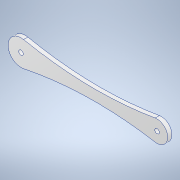
# Autodesk Inventor part: オムニ_支え板
Saved by Autodesk Inventor 2021 (Build 250183000, 183)
## iProperties
Created: 2022-02-03
Part Number: オムニ_支え板
Material: アルミニウム 6061
Document SubType Name: Modeling
Designer: hirohumi
Density: 2.7 g/cm^3
Appearance: アルミニウム - フラット
Author: hirohumi
Autodesk Inventor part; units mm, degrees
ref_plane "YZ Plane" through (0, 0, 0) normal (1, 0, 0) x (0, 1, 0)
ref_plane "XZ Plane" through (0, 0, 0) normal (0, 1, 0) x (-1, 0, 0)
ref_plane "XY Plane" through (0, 0, 0) normal (0, 0, 1) x (1, 0, 0)
sketch "スケッチ1" plane through (0, 0, 0) normal (0, 0, 1) x (1, 0, 0)
  circle A0 centre (-48, 0) radius 1.6
  circle A1 centre (48, 0) radius 1.6
  arc A2 (-46.163, 8.9126) -> (-46.163, -8.9126) centre (-48, 0) ccw
  arc A3 (46.7273, -7.3912) -> (46.7273, 7.3912) centre (48, 0) ccw
  arc A4 (-46.163, 8.9126) -> (46.7273, 7.3912) centre (4.305, 253.7656) ccw
  arc A5 (46.7273, -7.3912) -> (-46.163, -8.9126) centre (4.305, -253.7656) ccw
  point P0 (0, 0)
  dimension "d0" = 3.2
  dimension "d1" = 3.2
  dimension "d2" = 96
  dimension "d3" = 48
  dimension "d4" = 7.5
  dimension "d5" = 7.5
  dimension "d6" = 250
  dimension "d7" = 250
  constraints: 8 point on circle, 6 centre point, 4 tangent, 2 coincident, 2 horizontal alignment
  measures "d0" diameter of A0
  measures "d1" diameter of A1
  measures "d2" distance of A1.centre A0.centre
  measures "d3" distance of point (0, 0) A0.centre
  measures "d4" radial gap between concentric circles of A0 A2
  measures "d5" radius of A3
  measures "d6" radius of A4
  measures "d7" radius of A5
extrude "押し出し1" add sketch "スケッチ1" along normal blind 3
equation "\"d3\" = 0.5 * d2"
